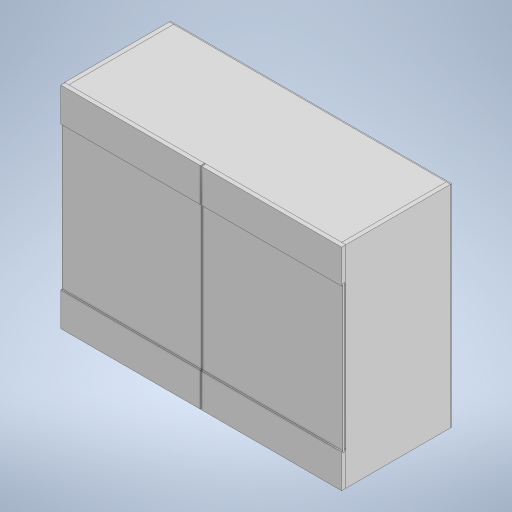
# Autodesk Inventor part: Wall Cabinet 3
Saved by Autodesk Inventor 2024 (Build 280153000, 153)
## iProperties
Created: 2023-06-24
Part Number: Wall Cabinet 3
Material: Generic
Document SubType Name: Modeling
Designer: 69
Density: 1 g/cm^3
Appearance: Default
Author: 69
Autodesk Inventor part; units mm, degrees
ref_plane "YZ Plane" through (0, 0, 0) normal (1, 0, 0) x (0, 1, 0)
sketch "Sketch1" plane through (0, 0, 0) normal (0, 0, 1) x (1, 0, 0)
  line L0 (-1498, 0) -> (1498, 0) construction
  line L1 (-1498, 0) -> (-898, 0)
  line L2 (-898, 0) -> (-898, 2068)
  line L3 (-898, 2068) -> (-1498, 2068)
  line L4 (-1498, 2068) -> (-1498, 0)
  line L5 (-898, 0) -> (-498, 0)
  line L6 (-498, 0) -> (-498, 816)
  line L7 (-498, 816) -> (-898, 816)
  line L8 (-898, 816) -> (-898, 0)
  line L9 (-498, 0) -> (102, 0)
  line L10 (102, 0) -> (102, 816)
  line L11 (102, 816) -> (-498, 816)
  line L12 (-498, 816) -> (-498, 0)
  line L13 (102, 0) -> (698, 0)
  line L14 (698, 0) -> (698, 668)
  line L15 (698, 668) -> (102, 668)
  line L16 (102, 668) -> (102, 0)
  line L17 (698, 0) -> (1498, 0)
  line L18 (1498, 0) -> (1498, 816)
  line L19 (1498, 816) -> (698, 816)
  line L20 (698, 816) -> (698, 0)
  line L21 (-1498, 0) -> (1498, 0)
  line L22 (1498, 0) -> (1498, 96)
  line L23 (1498, 96) -> (-1498, 96)
  line L24 (-1498, 96) -> (-1498, 0)
  line L25 (-898, 816) -> (1498, 816)
  line L26 (1498, 816) -> (1498, 832)
  line L27 (1498, 832) -> (-898, 832)
  line L28 (-898, 832) -> (-898, 816)
  line L29 (-898, 1972) -> (-498, 1972)
  line L30 (-498, 1972) -> (-498, 1372)
  line L31 (-498, 1372) -> (-898, 1372)
  line L32 (-898, 1372) -> (-898, 1972)
  line L33 (698, 1972) -> (1498, 1972)
  line L34 (1498, 1972) -> (1498, 1372)
  line L35 (1498, 1372) -> (698, 1372)
  line L36 (698, 1372) -> (698, 1972)
  line L37 (698, 1372) -> (98, 1372)
  line L38 (98, 1372) -> (98, 1972)
  line L39 (98, 1972) -> (698, 1972)
  line L40 (698, 1972) -> (698, 1372)
  line L41 (-498, 1372) -> (98, 1372)
  line L42 (-498, 1372) -> (-275, 1637.7611)
  line L43 (98, 1372) -> (-125, 1637.7611)
  line L44 (-275, 1637.7611) -> (-125, 1637.7611)
  line L45 (-125, 1637.7611) -> (-125, 2068)
  line L46 (-125, 2068) -> (-275, 2068)
  line L47 (-275, 2068) -> (-275, 1637.7611)
  line L48 (1098, 816) -> (1098, 96)
  line L49 (-198, 816) -> (-198, 96)
  line L50 (-898, 668) -> (-498, 668)
  line L51 (-1498, 520) -> (-898, 520)
  line L52 (-1498, 1579) -> (-898, 1579)
  line L53 (398, 1972) -> (398, 1372)
  line L54 (1098, 1972) -> (1098, 1372)
  line L55 (698, 1876) -> (1498, 1876)
  line L56 (698, 1468) -> (1498, 1468)
  line L57 (-1498, 1049.5) -> (-898, 1049.5)
  point P0 (0, 0)
  point P1 (0, 0)
  point P2 (0, 0)
  point P3 (-198, 816)
  point P4 (0, 0)
  dimension "d0" = 2996
  dimension "d1" = 600
  dimension "d2" = 2068
  dimension "d3" = 400
  dimension "d4" = 816
  dimension "d5" = 600
  dimension "d6" = 816
  dimension "d7" = 596
  dimension "d8" = 668
  dimension "d9" = 800
  dimension "d10" = 816
  dimension "d11" = 96
  dimension "d12" = 16
  dimension "d13" = 400
  dimension "d14" = 600
  dimension "d15" = 96
  dimension "d16" = 800
  dimension "d17" = 600
  dimension "d18" = 600
  dimension "d19" = 600
  dimension "d20" = 50
  dimension "d21" = 150
  dimension "d22" = 148
  dimension "d23" = 1059
  dimension "d24" = 96
  dimension "d25" = 96
  dimension "d26" = 529.5
  constraints: 116 end point, 22 parallel, 18 point on line, 17 perpendicular, 14 horizontal, 8 midpoint, 4 coincident, 4 horizontal alignment, 2 vertical alignment, 1 equal length
  measures "d0" distance of L0.start L0.end
  measures "d1" distance of L3.end L2.end
  measures "d2" distance of L2.end L1.end
  measures "d3" distance of L7.end L6.end
  measures "d4" distance of L6.end L5.end
  measures "d5" distance of L11.end L10.end
  measures "d6" distance of L9.end L10.end
  measures "d7" distance of L15.end L14.end
  measures "d8" distance of L14.end L13.end
  measures "d9" distance of L19.end L18.end
  measures "d10" distance of L18.end L17.end
  measures "d11" distance of L22.end L21.end
  measures "d12" distance of L26.end L25.end
  measures "d13" distance of L30.end L31.end
  measures "d14" distance of L29.end L30.end
  measures "d15" distance between parallel lines of L3 L29
  measures "d16" distance of L34.end L35.end
  measures "d17" distance of L33.end L34.end
  measures "d18" distance of L38.end L39.end
  measures "d19" distance of L37.end L38.end
  measures "d20" angle of L41 L42
  measures "d21" distance of L43.end L42.end
  measures "d22" distance of L50.start L51.end
  measures "d23" distance between parallel lines of L51 L52
  measures "d24" distance of L33.start L55.start
  measures "d25" distance of L56.start L35.end
  measures "d26" distance between parallel lines of L51 L57
ref_plane "Work Plane1" through (1498, 1372, 0) normal (0, 1, 0) x (-1, 0, 0)
sketch "Sketch2" plane through (1498, 1372, 0) normal (0, 1, 0) x (-1, 0, 0)
  line L0 (800, 0) -> (0, 0)
  line L1 (0, 0) -> (0, 310)
  line L2 (0, 310) -> (800, 310)
  line L3 (800, 310) -> (800, 0)
  line L4 (788, 298) -> (12, 298)
  line L5 (12, 298) -> (12, 12)
  line L6 (12, 12) -> (788, 12)
  line L7 (788, 12) -> (788, 298)
  line L8 (788, 12) -> (788, 0)
  line L9 (12, 12) -> (12, 0)
  line L10 (12, 298) -> (0, 298)
  line L11 (788, 298) -> (800, 298)
  point P0 (1498, 0)
  point P1 (0, 0)
  point P2 (0, 0)
  point P3 (0, 0)
  point P4 (800, 0)
  dimension "d28" = 800
  dimension "d29" = 310
  dimension "d30" = 12
  constraints: 24 end point, 5 point on line, 4 parallel, 4 perpendicular, 1 horizontal, 1 vertical, 3 other
  measures "d28" distance of L1.end L2.end
  measures "d29" distance of L0.end L1.end
  measures "d30" distance between parallel lines of L2 L4
extrude "Extrusion1" add sketch "Sketch2" along normal up to surface (600 mm away) contours L0 L8 L7 L11 L3 | L0 L1 L10 L5 L9
extrude "Extrusion2" add sketch "Sketch2" along normal up to surface (600 mm away) separate body contours L11 L4 L10 L1 L2 L3
split body "Split1" sketch "Sketch1" result two bodies bodies 2 curves L54 first body at (1231.3333, 1572, 309.5)
sketch "Sketch3" plane through (1498, 1372, 0) normal (0, 1, 0) x (-1, 0, 0)
  line L0 (800, 0) -> (788, 0) projected
  line L1 (800, 0) -> (0, 0)
  line L2 (0, 0) -> (0, -3)
  line L3 (0, -3) -> (800, -3)
  line L4 (800, -3) -> (800, 0)
  point P0 (1498, 0)
  dimension "d35" = 3
  constraints: 8 end point, 2 parallel, 1 coincident, 1 horizontal, 1 perpendicular
  measures "d35" distance of L1.end L2.end
extrude "Extrusion3" add sketch "Sketch3" along normal up to surface (600 mm away) separate body
split body "Split2" sketch "Sketch1" result two bodies bodies 4 curves L55 first body at (831.3333, 1908, 309.5)
split body "Split3" sketch "Sketch1" result one side removed bodies 7 curves L56 removed pieces at (831.3333, 1604, 309.5)
split body "Split4" sketch "Sketch1" result two bodies bodies 3 curves L55 first body at (1231.3333, 1908, 309.5)
split body "Split5" sketch "Sketch1" result one side removed bodies 9 curves L56 removed pieces at (1231.3333, 1604, 309.5)
sketch "Sketch4" plane through (1498, 1372, 0) normal (0, 1, 0) x (-1, 0, 0)
  line L0 (788, 0) -> (788, 298) projected
  line L1 (0, 0) -> (800, 0) projected
  line L2 (12, 298) -> (12, 0) projected
  line L3 (400, 298) -> (0, 298) projected
  line L4 (800, 298) -> (400, 298) projected
  point P0 (1498, 0)
extrude "Extrusion4" add sketch "Sketch4" along normal blind 12 separate body
ref_plane "Work Plane2" through (1498, 1972, 223.5) normal (0, -1, 0) x (0, 0, 1)
sketch "Sketch5" plane through (1498, 1972, 223.5) normal (0, -1, 0) x (0, 0, 1)
  line L0 (-223.5, 0) -> (-223.5, 800) projected
  line L1 (-223.5, 788) -> (74.5, 788) projected
  line L2 (74.5, 12) -> (-223.5, 12) projected
  line L3 (74.5, 400) -> (74.5, 0) projected
  line L4 (74.5, 800) -> (74.5, 400) projected
  point P0 (-223.5, 1498)
extrude "Extrusion5" add sketch "Sketch5" along normal blind 12 separate body
sketch "Sketch6" plane through (1498, 1372, 298) normal (1, 0, 0) x (0, 0, -1)
  line L0 (0, 0) -> (0, 600) projected
  line L1 (0, 300) -> (388.0089, 300) construction
  line L2 (-8.5, 504) -> (-3.5, 504)
  line L3 (-3.5, 504) -> (-3.5, 509)
  line L4 (-3.5, 509) -> (-8.5, 509)
  line L5 (-8.5, 509) -> (-8.5, 504)
  line L6 (0, 504) -> (-12, 504) projected
  line L7 (-8.5, 96) -> (-3.5, 96)
  line L8 (-3.5, 96) -> (-3.5, 91)
  line L9 (-3.5, 91) -> (-8.5, 91)
  line L10 (-8.5, 91) -> (-8.5, 96)
  point P0 (298, -1372)
  point P1 (-6, 504)
  dimension "d42" = 5
  dimension "d43" = 5
  constraints: 18 end point, 4 symmetric about line, 3 midpoint, 2 horizontal, 2 parallel, 1 perpendicular
  measures "d42" distance of L3.end L4.end
  measures "d43" distance of L4.end L2.start
extrude "Extrusion6" cut sketch "Sketch6" against normal blind 900 contours L5 L4 L3 L2 bodies 8
extrude "Extrusion7" cut sketch "Sketch6" against normal blind 900 contours L5 L4 L3 L2 bodies 6
extrude "Extrusion8" cut sketch "Sketch6" against normal blind 900 contours L7 L8 L9 L10 bodies 1 9
extrude "Extrusion9" cut sketch "Sketch6" against normal blind 900 contours L7 L8 L9 L10 bodies 7
sketch "Sketch7" plane through (1498, 1372, 298) normal (1, 0, 0) x (0, 0, -1)
  line L0 (-8.5, 509) -> (-8.5, 504) projected
  line L1 (-3.5, 91) -> (-8.5, 91) projected
  line L2 (-8.5, 509) -> (-3.5, 509)
  line L3 (-3.5, 509) -> (-3.5, 91)
  line L4 (-3.5, 91) -> (-8.5, 91)
  line L5 (-8.5, 91) -> (-8.5, 509)
  point P0 (298, -1372)
  constraints: 8 end point, 2 parallel, 1 horizontal, 1 perpendicular
extrude "Extrusion10" add sketch "Sketch7" against normal up to surface (800 mm away) separate body
split body "Split6" sketch "Sketch1" result two bodies bodies 12 curves L54 first body at (1231.3333, 1602.3333, 302)
sketch "Sketch8" plane through (698, 1972, 310) normal (0, 0, 1) x (1, 0, 0)
  line L0 (12, 0) -> (788, 0) projected
  line L1 (12, -600) -> (788, -600) projected
  line L2 (398.5, 0) -> (401.5, 0)
  line L3 (401.5, 0) -> (401.5, -600)
  line L4 (401.5, -600) -> (398.5, -600)
  line L5 (398.5, -600) -> (398.5, 0)
  line L6 (400, -96) -> (400, 0) projected
  point P0 (-698, -1972)
  point P1 (398.5, -600)
  point P2 (401.5, 0)
  dimension "d54" = 1.5
  dimension "d55" = 1.5
  constraints: 8 end point, 2 parallel, 2 point on line, 1 horizontal, 1 perpendicular
  measures "d54" distance between parallel lines of L6 L3
  measures "d55" distance between parallel lines of L6 L5
extrude "Extrusion11" cut sketch "Sketch8" against normal blind 12 bodies 6 14 7 9 13 8
sketch "Sketch9" plane through (698, 1372, 0) normal (0, 0, 1) x (1, 0, 0)
  line L0 (12, 0) -> (12, 600) projected
  line L1 (788, 0) -> (788, 600) projected
  line L2 (12, 306) -> (788, 306)
  line L3 (788, 306) -> (788, 294)
  line L4 (788, 294) -> (12, 294)
  line L5 (12, 294) -> (12, 306)
  line L6 (12, 12) -> (788, 12) projected
  point P0 (-698, -1372)
  point P1 (12, 294)
  point P2 (788, 306)
  dimension "d58" = 282
  dimension "d59" = 12
  constraints: 8 end point, 2 parallel, 2 point on line, 1 horizontal, 1 perpendicular
  measures "d58" distance between parallel lines of L6 L4
  measures "d59" distance between parallel lines of L4 L2
extrude "Extrusion12" add sketch "Sketch9" along normal up to surface (298 mm away) separate body contours L0 L2 L1 L4
sketch "Sketch10" plane through (698, 1876, 310) normal (0, 0, 1) x (1, 0, 0)
  line L0 (800, -504) -> (0, -504) projected
  line L1 (0, 96) -> (1.5, 96)
  line L2 (1.5, 96) -> (1.5, -504)
  line L3 (1.5, -504) -> (0, -504)
  line L4 (0, -504) -> (0, 96)
  line L5 (0, -413) -> (0, 5) projected
  point P0 (-698, -1876)
  dimension "d62" = 1.5
  constraints: 8 end point, 2 parallel, 1 horizontal, 1 perpendicular, 1 point on line
  measures "d62" distance between parallel lines of L2 L5
extrude "Extrusion13" cut sketch "Sketch10" against normal blind 12 bodies 6 7 14
